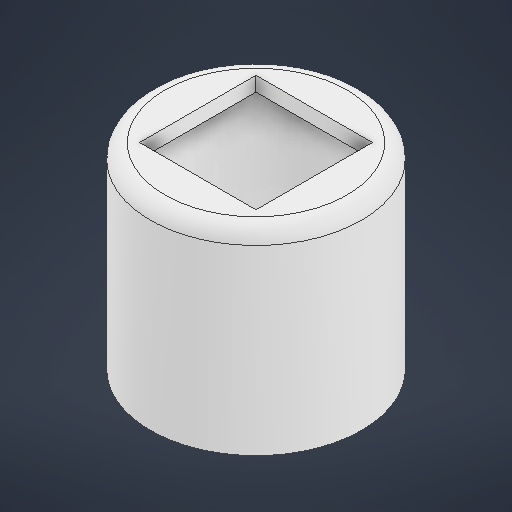
# Autodesk Inventor part: module
Saved by Autodesk Inventor 2026.2 (Build 302298000, 298)
## iProperties
Created: 2026-04-08
Part Number: module
Material: ABS Plastic
Document SubType Name: Modeling
Designer: Koda
Density: 1.06 g/cm^3
Appearance: Smooth - White
Author: Koda
Autodesk Inventor part; units mm, degrees
ref_plane "YZ Plane" through (0, 0, 0) normal (1, 0, 0) x (0, 1, 0)
ref_plane "XZ Plane" through (0, 0, 0) normal (0, 1, 0) x (-1, 0, 0)
ref_plane "XY Plane" through (0, 0, 0) normal (0, 0, 1) x (1, 0, 0)
sketch "Sketch1" plane through (0, 0, 0) normal (0, 1, 0) x (-1, 0, 0)
  circle A0 centre (0, 0) radius 18.415
  dimension "d0" = 36.83
  constraints: 1 centre point, 1 coincident
  measures "d0" diameter of A0
extrude "Extrusion1" add sketch "Sketch1" along normal blind 34.29
fillet "Fillet1" radius 2.54 1 edges at (18.415, 34.29, 0)
sketch "Sketch2" plane through (0, 0, 0) normal (0, -1, 0) x (1, 0, 0)
  circle A0 centre (0, 0) radius 15.24
  dimension "d4" = 30.48
  constraints: 1 centre point, 1 coincident
  measures "d4" diameter of A0
extrude "Extrusion2" cut sketch "Sketch2" against normal blind 31.75
sketch "Sketch3" plane through (0, 34.29, 0) normal (0, 1, 0) x (1, 0, 0)
  line L0 (0, 0) -> (0, -10.16)
  line L1 (0, 0) -> (-10.16, 0)
  line L2 (-10.16, -10.16) -> (10.16, -10.16)
  line L3 (10.16, -10.16) -> (10.16, 10.16)
  line L4 (10.16, 10.16) -> (-10.16, 10.16)
  line L5 (-10.16, 10.16) -> (-10.16, -10.16)
  dimension "d7" = 10.16
  dimension "d8" = 10.16
  dimension "d9" = 20.32
  dimension "d10" = 20.32
  constraints: 12 end point, 2 horizontal, 2 parallel, 1 perpendicular, 1 vertical
  measures "d7" distance of L0.start L0.end
  measures "d8" distance of L0.start L1.end
  measures "d9" distance of L4.end L3.end
  measures "d10" distance of L3.end L2.end
extrude "Extrusion3" cut sketch "Sketch3" against normal blind 31.75
sketch "Sketch4" plane through (0, 0, 0) normal (0, -1, 0) x (1, 0, 0)
  line L0 (10.16, 10.16) -> (-10.16, 10.16) projected
  line L1 (0, 10.16) -> (-11.3592, 10.16)
  circle A0 centre (0, 0) radius 15.24 projected
  line L2 (0, 10.16) -> (11.3592, 10.16)
  circle A1 centre (0, 0) radius 15.24
  constraints: 4 end point, 2 point on circle, 1 centre point, 1 coincident, 1 concentric, 1 horizontal, 1 midpoint, 1 point on line
extrude "Extrusion4" add sketch "Sketch4" against normal blind 34.29 contours L0 L1 A0 L2 picked at (-6.2582, 10.9638)
body "Solid1"
